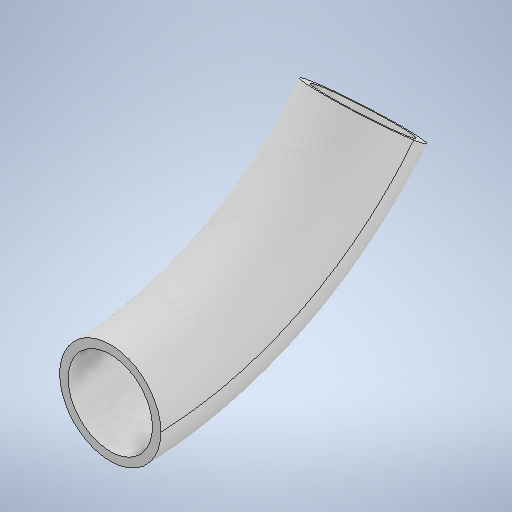
# Autodesk Inventor part: Sweep
Saved by Autodesk Inventor 2025.2 (Build 292293000, 293)
## iProperties
Created: 2025-03-25
Part Number: Sweep
Material: Generic
Document SubType Name: Modeling
Designer: ishad
Density: 1 g/cm^3
Appearance: Default
Author: ishad
Autodesk Inventor part; units mm, degrees
ref_plane "YZ Plane" through (0, 0, 0) normal (1, 0, 0) x (0, 1, 0)
ref_plane "XZ Plane" through (0, 0, 0) normal (0, 1, 0) x (-1, 0, 0)
ref_plane "XY Plane" through (0, 0, 0) normal (0, 0, 1) x (1, 0, 0)
sketch "Sketch1" plane through (0, 0, 0) normal (0, 0, 1) x (1, 0, 0)
  circle A0 centre (0, 0) radius 6
  circle A1 centre (0, 0) radius 5
  dimension "d12" = 10
  dimension "d13" = 1
  constraints: 2 centre point, 2 coincident
  measures "d12" diameter of A1
  measures "d13" radial gap between concentric circles of A1 A0
sketch "Sketch2" plane through (0, 0, 0) normal (1, 0, 0) x (0, 1, 0)
  arc A0 (0, 0) -> (15, -30) centre (39.9808, 1.2404) ccw
  dimension "d7" = 15
  dimension "d8" = 40
  dimension "d9" = 30
  constraints: 2 point on circle, 1 centre point, 1 coincident
  measures "d7" horizontal distance of point (0, 0) A0.end
  measures "d8" radius of A0
  measures "d9" vertical distance of point (0, 0) A0.end
sweep "Sweep1" add profiles "Sketch1" path "Sketch2"
body "Solid1"
